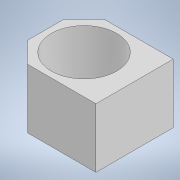
# Autodesk Inventor part: OsnovaBaraban
Saved by Autodesk Inventor 2022 (Build 260153000, 153)
## iProperties
Created: 2023-08-16
Part Number: OsnovaBaraban
Material: Generic
Document SubType Name: Modeling
Designer: Kippi
Density: 1 g/cm^3
Appearance: Default
Author: Kippi
Autodesk Inventor part; units mm, degrees
ref_plane "YZ Plane" through (0, 0, 0) normal (1, 0, 0) x (0, 1, 0)
ref_plane "XZ Plane" through (0, 0, 0) normal (0, 1, 0) x (-1, 0, 0)
ref_plane "XY Plane" through (0, 0, 0) normal (0, 0, 1) x (1, 0, 0)
sketch "Sketch1" plane through (0, 0, 0) normal (0, 1, 0) x (-1, 0, 0)
  line L0 (54.5455, 79) -> (-95.4545, 79)
  line L1 (-95.4545, 79) -> (-95.4545, -51)
  line L2 (-95.4545, -51) -> (54.5455, -51)
  line L3 (54.5455, -51) -> (54.5455, 79)
  circle A0 centre (-10.4545, 14) radius 55
  line L4 (54.5455, -16) -> (19.5455, -51)
  line L5 (54.5455, 44) -> (19.5455, 79)
  point P0 (0, 0)
  dimension "d0" = 130
  dimension "d1" = 35
  dimension "d2" = 35
  dimension "d3" = 35
  dimension "d4" = 35
  dimension "d5" = 65
  dimension "d6" = 110
  dimension "d7" = 65
  dimension "d10" = 150
  constraints: 12 end point, 4 point on line, 2 parallel, 2 perpendicular, 1 centre point, 1 horizontal
  measures "d0" distance of L2.end L0.start
  measures "d1" distance of L2.end L4.start
  measures "d2" distance of L2.end L4.end
  measures "d3" distance of L0.start L5.start
  measures "d4" distance of L0.start L5.end
  measures "d5" distance from line of L0 A0.centre
  measures "d6" diameter of A0
  measures "d7" distance from line of L3 A0.centre
  measures "d10" distance of L0.start L0.end
extrude "Extrusion1" add sketch "Sketch1" along normal blind 100 contours L5 L3 L4 L2 L1 L0
body "Solid1"
